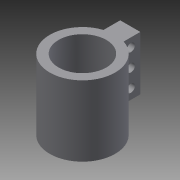
# Autodesk Inventor part: brush holder v5
Saved by Autodesk Inventor 2013 SP2 (Build 170200200, 200)
## iProperties
Created: 2017-05-15
Part Number: brush holder v5
Material: Generic
Document SubType Name: Modeling
Designer: Herman de Vries
Density: 1 g/cm^3
Author: Herman de Vries
Autodesk Inventor part; units mm, degrees
ref_plane "YZ Plane" through (0, 0, 0) normal (1, 0, 0) x (0, 1, 0)
ref_plane "XZ Plane" through (0, 0, 0) normal (0, 1, 0) x (-1, 0, 0)
ref_plane "XY Plane" through (0, 0, 0) normal (0, 0, 1) x (1, 0, 0)
sketch "Sketch1" plane through (0, 0, 0) normal (1, 0, 0) x (0, 1, 0)
  line L0 (0, 12.5) -> (0, 0) construction
  line L1 (13, 0) -> (13, 28)
  line L2 (13, 28) -> (9.5, 28)
  line L3 (9.5, 28) -> (10.4778, 0)
  line L4 (13, 0) -> (10.4778, 0)
  dimension "d36" = 13
  dimension "d63" = 28
  dimension "d65" = 9.5
  dimension "d66" = 92
  constraints: 11 end point, 2 horizontal, 2 vertical, 1 horizontal alignment
  measures "d36" distance from line of L1 L0.end
  measures "d63" distance of L1.start L1.end
  measures "d65" distance from line of L0 L2.end
  measures "d66" angle of L4 L3
revolve "Revolution1" add sketch "Sketch1" angle 360 about axis through (0, 0, 12.5) along (0, 0, -1)
sketch "Sketch3" plane through (0, 0, 0) normal (1, 0, 0) x (0, 1, 0)
  line L0 (19, 0) -> (19, 28)
  line L1 (19, 28) -> (10.4778, 28)
  line L2 (19, 0) -> (10.4778, 0)
  line L3 (-10.4778, 0) -> (10.4778, 0) projected
  line L4 (10.4778, 0) -> (10.4778, 28)
  line L5 (-13, 28) -> (13, 28) projected
  point P0 (0, 0)
  dimension "d28" = 19
  constraints: 8 end point, 2 vertical, 1 collinear, 1 horizontal
  measures "d28" distance from line of L0 point (0, 0)
extrude "Extrusion1" add sketch "Sketch3" along normal mid plane 8
sketch "Sketch4" plane through (-4, 0, 0) normal (-1, 0, 0) x (0, 0, 1)
  circle A0 centre (10.5, 15.25) radius 1.6
  circle A1 centre (17.5, 15.25) radius 1.6
  line L0 (10.5, 15.25) -> (17.5, 15.25) construction
  line L1 (28, 19) -> (0, 19) construction
  circle A2 centre (24.5, 15.25) radius 1.6
  point P0 (0, 0)
  point P1 (17, 15.25)
  point P2 (14, 15.25)
  point P3 (14, 19)
  dimension "d29" = 3.2
  dimension "d30" = 3.2
  dimension "d31" = 7
  dimension "d34" = 3.75
  dimension "d67" = 3.2
  dimension "d68" = 7
  constraints: 3 centre point, 3 horizontal alignment, 2 end point, 2 midpoint, 1 horizontal, 1 vertical alignment
  measures "d29" diameter of A0
  measures "d30" diameter of A1
  measures "d31" distance of L0.start L0.end
  measures "d34" distance between parallel lines of L0 L1
  measures "d67" diameter of A2
  measures "d68" distance of A2.centre L0.end
extrude "Extrusion2" cut sketch "Sketch4" against normal blind 10
sketch "Sketch5" plane through (4, 0, 0) normal (1, 0, 0) x (0, 0, -1)
  circle A0 centre (-10.5, 15.25) radius 1.6 projected
  circle A1 centre (-17.5, 15.25) radius 1.6 projected
  line L0 (0, 12.3693) -> (-28, 12.3693) projected
  line L1 (-20.496, 19) -> (-21.5, 19)
  line L2 (-21.5, 19) -> (-21.5, 12.3693)
  line L3 (-21.5, 12.3693) -> (-20.496, 12.3693)
  line L4 (-20.496, 12.3693) -> (-20.496, 19)
  line L5 (0, 19) -> (-6.5, 19)
  line L6 (-6.5, 19) -> (-6.5, 12.3693)
  line L7 (-6.5, 12.3693) -> (0, 12.3693)
  line L8 (0, 12.3693) -> (0, 19)
  line L9 (0, 19) -> (-28, 19) projected
  point P0 (0, 0)
  dimension "d47" = 15
  dimension "d49" = 4
  dimension "d50" = 4
  constraints: 16 end point, 4 parallel, 2 horizontal, 2 perpendicular, 2 point on line, 1 collinear
  measures "d47" distance between parallel lines of L6 L2
  measures "d49" distance from line of L2 A1.centre
  measures "d50" distance from line of L6 A0.centre
extrude "Extrusion3" cut sketch "Sketch5" against normal blind 10 contours L0 L6 L5 L8
equation "\"d49\" = d50"
body "Solid1"
